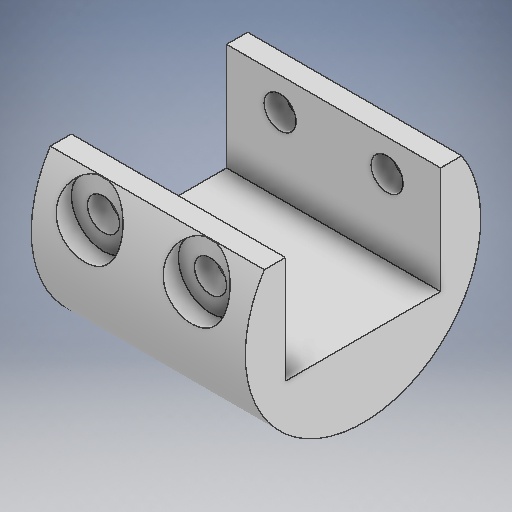
# Autodesk Inventor part: shoe
Saved by Autodesk Inventor 2026.1 (Build 301233000, 233)
## iProperties
Created: 2025-12-16
Part Number: shoe
Material: Generic
Document SubType Name: Modeling
Designer: emanuel
Density: 1 g/cm^3
Appearance: Default
Author: emanuel
Autodesk Inventor part; units mm, degrees
ref_plane "YZ Plane" through (0, 0, 0) normal (1, 0, 0) x (0, 1, 0)
ref_plane "XZ Plane" through (0, 0, 0) normal (0, 1, 0) x (-1, 0, 0)
ref_plane "XY Plane" through (0, 0, 0) normal (0, 0, 1) x (1, 0, 0)
sketch "Sketch1" plane through (0, 0, 0) normal (1, 0, 0) x (0, 1, 0)
  circle A0 centre (0, 0) radius 11
  line L0 (0, 0) -> (0, -7.25)
  line L1 (0, 0) -> (0, 7.25)
  line L2 (0, 7.25) -> (6, 7.25)
  line L3 (6, 7.25) -> (6, 10)
  line L4 (6, 10) -> (0, 10)
  line L5 (0, 10) -> (0, 7.25)
  line L6 (0, -7.25) -> (6, -7.25)
  line L7 (6, -7.25) -> (6, -10)
  line L8 (6, -10) -> (0, -10)
  line L9 (0, -10) -> (0, -7.25)
  line L10 (0, 7.25) -> (-4, 7.25)
  line L11 (-4, 7.25) -> (-4, -7.25)
  line L12 (-4, -7.25) -> (0, -7.25)
  line L13 (0, -7.25) -> (0, 7.25)
  point P0 (6, 9.2195)
  point P1 (6, -9.2195)
  dimension "d0" = 22
  dimension "d1" = 7.25
  dimension "d2" = 7.25
  dimension "d3" = 6
  dimension "d4" = 4
  constraints: 28 end point, 6 parallel, 3 horizontal, 3 perpendicular, 2 vertical, 1 centre point, 1 coincident, 1 point on line
  measures "d0" diameter of A0
  measures "d1" distance of L0.start L0.end
  measures "d2" distance of L0.start L1.end
  measures "d3" distance of L4.end L3.end
  measures "d4" distance of L12.end L11.end
extrude "Extrusion1" add sketch "Sketch1" along normal blind 20 contours L3 L2 L5 L4 A0 | A0 L8 L9 L6 L7 | L4 L5 L10 L11 L12 L9 L8 A0
sketch "Sketch2" plane through (0, -4, -7.25) normal (0, 0, 1) x (1, 0, 0)
  line L0 (0, 10) -> (20, 10) projected
  line L1 (0, 10) -> (5, 10)
  line L2 (5, 10) -> (5, 7)
  line L3 (5, 7) -> (0, 7)
  line L4 (0, 7) -> (0, 10)
  line L5 (20, 10) -> (15, 10)
  line L6 (15, 10) -> (15, 7)
  line L7 (15, 7) -> (20, 7)
  line L8 (20, 7) -> (20, 10)
  circle A0 centre (15, 7) radius 1.5
  circle A1 centre (5, 7) radius 1.5
  point P0 (0, 4)
  dimension "d7" = 5
  dimension "d8" = 3
  dimension "d9" = 5
  dimension "d10" = 3
  dimension "d11" = 3
  dimension "d12" = 3
  constraints: 16 end point, 4 parallel, 2 centre point, 2 coincident, 2 horizontal, 2 perpendicular
  measures "d7" distance of L2.end L3.end
  measures "d8" distance of L1.end L2.end
  measures "d9" distance of L7.end L6.end
  measures "d10" distance of L6.end L5.end
  measures "d11" diameter of A0
  measures "d12" diameter of A1
extrude "Extrusion2" cut sketch "Sketch2" along normal mid plane 50 contours A1 L3 L2 | L2 L3 A1 | A0 L7 L6 | L6 L7 A0
ref_plane "Work Plane1" through (0, -4, -17.25) normal (0, 0, 1) x (1, 0, 0)
sketch "Sketch3" plane through (0, -4, -17.25) normal (0, 0, 1) x (1, 0, 0)
  circle A0 centre (15, 7) radius 1.5 projected
  circle A1 centre (15, 7) radius 3
  circle A2 centre (5, 7) radius 1.5 projected
  circle A3 centre (5, 7) radius 3
  point P0 (0, 4)
  dimension "d16" = 6
  dimension "d17" = 6
  constraints: 2 centre point, 2 coincident
  measures "d16" diameter of A1
  measures "d17" diameter of A3
extrude "Extrusion3" cut sketch "Sketch3" along normal blind 8
ref_plane "Work Plane2" through (0, -4, 17.25) normal (0, 0, -1) x (-1, 0, 0)
sketch "Sketch4" plane through (0, -4, 17.25) normal (0, 0, -1) x (-1, 0, 0)
  circle A0 centre (-5, 7) radius 1.5 projected
  circle A1 centre (-5, 7) radius 3
  line L0 (0, 10) -> (-20, 10) projected
  circle A2 centre (-15, 7) radius 1.5 projected
  circle A3 centre (-15, 7) radius 3
  point P0 (0, 4)
  point P1 (-15.0159, 10)
  point P2 (-14.9841, 10)
  constraints: 2 centre point, 2 coincident, 1 tangent
extrude "Extrusion4" cut sketch "Sketch4" along normal blind 8
body "Solid1"
